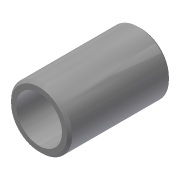
# Autodesk Inventor part: Coupler
Saved by Autodesk Inventor 2021 (Build 250183000, 183)
## iProperties
Created: 2013-05-06
Part Number: Coupler
Material: Steel, Mild
Document SubType Name: Modeling
Designer: user
Mass: 2522.6 g
Surface Area: 556.927 cm^2
Volume: 320.941 cm^3
Density: 7.86 g/cm^3
Appearance: Steel
Author: user
Autodesk Inventor part; units mm, degrees
ref_plane "YZ Plane" through (0, 0, 0) normal (1, 0, 0) x (0, 1, 0)
ref_plane "XZ Plane" through (0, 0, 0) normal (0, 1, 0) x (-1, 0, 0)
ref_plane "XY Plane" through (0, 0, 0) normal (0, 0, 1) x (1, 0, 0)
sketch "Sketch1" plane through (0, 0, 0) normal (0, 0, 1) x (1, 0, 0)
  circle A0 centre (0, 0) radius 38.1
  dimension "d0" = 76.2
  constraints: 1 centre point, 1 coincident
  measures "d0" diameter of A0
extrude "Extrusion1" add sketch "Sketch1" along normal blind 127
chamfer "Chamfer1" distance 3.175 angle 45 2 edges at (-38.1, 0, 0) (-38.1, 0, 127)
sketch "Sketch2" plane through (0, 0, 127) normal (0, 0, 1) x (1, 0, 0)
  point P0 (0, 0)
hole "Hole1" at (0, 0, 127) direction (0, 0, -1) diameter 43.18 end through all counterbore diameter 57.15 counterbore depth 63.5 clearance for "Hex Head Bolt" size "1-1/2" standard "Ansi Unified Screw Threads"
body "Solid1"
